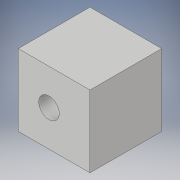
# Autodesk Inventor part: CLB_078_ScissorBottomBarPlug
Saved by Autodesk Inventor 2018.3 (Build 223284000, 284)
## iProperties
Created: 2020-02-18
Part Number: CLB_078_ScissorBottomBarPlug
Material: Generic
Document SubType Name: Modeling
Designer: 22perngrac
Density: 1 g/cm^3
Appearance: Default
Author: 22perngrac
Autodesk Inventor part; units mm, degrees
ref_plane "YZ Plane" through (0, 0, 0) normal (1, 0, 0) x (0, 1, 0)
ref_plane "XZ Plane" through (0, 0, 0) normal (0, 1, 0) x (-1, 0, 0)
ref_plane "XY Plane" through (0, 0, 0) normal (0, 0, 1) x (1, 0, 0)
sketch "Sketch1" plane through (0, 0, 0) normal (0, 0, 1) x (1, 0, 0)
  line L0 (0, 0) -> (22.225, 0)
  line L1 (22.225, 0) -> (22.225, 22.225)
  line L2 (22.225, 22.225) -> (0, 22.225)
  line L3 (0, 22.225) -> (0, 0)
  dimension "d21" = 22.225
  dimension "d22" = 22.225
  constraints: 8 end point, 2 parallel, 1 horizontal, 1 perpendicular
  measures "d21" distance of L1.end L2.end
  measures "d22" distance of L0.end L1.end
extrude "Extrusion1" add sketch "Sketch1" along normal blind 22.225
sketch "Sketch5" plane through (0, 0, 22.225) normal (0, 0, 1) x (1, 0, 0)
  line L0 (22.225, 0) -> (22.225, 22.225) projected
  line L1 (22.225, 22.225) -> (0, 22.225) projected
  point P0 (0, 0)
  point P1 (9.525, 11.1125)
  dimension "d33" = 12.7
  dimension "d34" = 11.1125
  measures "d33" distance from line of point (9.525, 11.113) L0
  measures "d34" distance from line of L1 point (9.525, 11.113)
hole "Hole4" at (9.525, 11.1125, 22.225) direction (0, 0, -1) diameter 6.35 end through all
body "Solid1"
